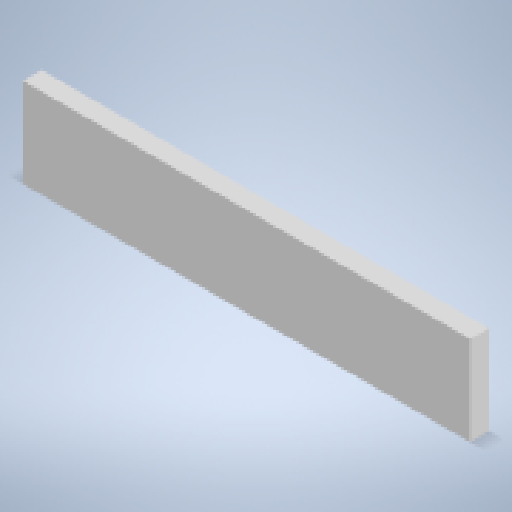
# Autodesk Inventor part: Matrices
Saved by Autodesk Inventor 2024 (Build 280153000, 153)
## iProperties
Created: 2024-01-06
Part Number: Matrices
Material: Genérico
Document SubType Name: Modeling
Designer: sergi
Density: 1 g/cm^3
Appearance: Valor por defecto
Author: sergi
Autodesk Inventor part; units mm, degrees
ref_plane "YZ Plane" through (0, 0, 0) normal (1, 0, 0) x (0, 1, 0)
ref_plane "XZ Plane" through (0, 0, 0) normal (0, 1, 0) x (-1, 0, 0)
ref_plane "XY Plane" through (0, 0, 0) normal (0, 0, 1) x (1, 0, 0)
sketch "Boceto1" plane through (0, 0, 0) normal (0, 0, 1) x (1, 0, 0)
  line L0 (-129.86, -38.51) -> (-129.86, -45.51) projected
  line L1 (-129.86, -45.51) -> (39.14, -45.51) projected
  arc A0 (39.14, -45.51) -> (39.64, -45.01) centre (39.14, -45.01) ccw projected
  line L2 (39.64, -45.01) -> (39.64, 32.69) projected
  arc A1 (39.64, 32.69) -> (39.14, 33.19) centre (39.14, 32.69) ccw projected
  line L3 (39.14, 33.19) -> (-129.86, 33.19) projected
  line L4 (-129.86, 33.19) -> (-129.86, 26.19) projected
  line L5 (-129.86, 26.19) -> (32.64, 26.19) projected
  line L6 (32.64, 26.19) -> (32.64, -38.51) projected
  line L7 (32.64, -38.51) -> (-129.86, -38.51) projected
  circle A2 centre (36.14, 29.69) radius 2.15 projected
  circle A3 centre (36.14, -42.01) radius 2.15 projected
  circle A4 centre (-74.5267, 29.69) radius 2.15 projected
  circle A5 centre (-74.5267, -42.01) radius 2.15 projected
  line L8 (-129.86, -45.51) -> (-129.86, -38.51) projected
  line L9 (-129.86, -38.51) -> (-292.36, -38.51) projected
  line L10 (-292.36, -38.51) -> (-292.36, 26.19) projected
  line L11 (-292.36, 26.19) -> (-129.86, 26.19) projected
  line L12 (-129.86, 26.19) -> (-129.86, 33.19) projected
  line L13 (-129.86, 33.19) -> (-298.86, 33.19) projected
  arc A6 (-298.86, 33.19) -> (-299.36, 32.69) centre (-298.86, 32.69) ccw projected
  line L14 (-299.36, 32.69) -> (-299.36, -45.01) projected
  arc A7 (-299.36, -45.01) -> (-298.86, -45.51) centre (-298.86, -45.01) ccw projected
  line L15 (-298.86, -45.51) -> (-129.86, -45.51) projected
  circle A8 centre (-185.1933, 29.69) radius 2.15 projected
  circle A9 centre (-295.86, -42.01) radius 2.15 projected
  circle A10 centre (-295.86, 29.69) radius 2.15 projected
  circle A11 centre (-185.1933, -42.01) radius 2.15 projected
  line L16 (32.64, -38.51) -> (-292.36, -38.51)
  line L17 (-292.36, -38.51) -> (-292.36, 26.19)
  line L18 (-292.36, 26.19) -> (32.64, 26.19)
  line L19 (32.64, 26.19) -> (32.64, -38.51)
  point P0 (0, 0)
  constraints: 8 end point, 2 parallel, 1 horizontal, 1 perpendicular
extrude "Extrusión1" add sketch "Boceto1" along normal blind 13.7 contours L9 L10 L11 L5 L6 L7
